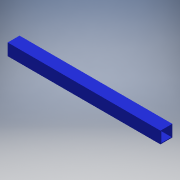
# Autodesk Inventor part: cross brace
Saved by Autodesk Inventor 2017 SP1 (Build 210196100, 196)
## iProperties
Created: 2018-01-26
Part Number: cross brace
Material: Aluminum 6061
Document SubType Name: Modeling
Designer: Ben
Density: 2.7 g/cm^3
Appearance: Blue - Wall Paint - Glossy
Author: Ben
Autodesk Inventor part; units mm, degrees
ref_plane "YZ Plane" through (0, 0, 0) normal (1, 0, 0) x (0, 1, 0)
ref_plane "XZ Plane" through (0, 0, 0) normal (0, 1, 0) x (-1, 0, 0)
ref_plane "XY Plane" through (0, 0, 0) normal (0, 0, 1) x (1, 0, 0)
sketch "Sketch1" plane through (0, 0, 0) normal (1, 0, 0) x (0, 1, 0)
  line L0 (-12.7, 12.7) -> (12.7, 12.7)
  line L1 (12.7, 12.7) -> (12.7, -12.7)
  line L2 (12.7, -12.7) -> (-12.7, -12.7)
  line L3 (-12.7, -12.7) -> (-12.7, 12.7)
  line L4 (-12.7, 12.7) -> (12.7, -12.7) construction
  line L5 (12.7, 12.7) -> (-12.7, -12.7) construction
  line L6 (-11.1125, 11.1125) -> (11.1125, 11.1125)
  line L7 (11.1125, 11.1125) -> (11.1125, -11.1125)
  line L8 (11.1125, -11.1125) -> (-11.1125, -11.1125)
  line L9 (-11.1125, -11.1125) -> (-11.1125, 11.1125)
  line L10 (-11.1125, 11.1125) -> (11.1125, -11.1125) construction
  line L11 (11.1125, 11.1125) -> (-11.1125, -11.1125) construction
  point P0 (0, 0)
  dimension "d0" = 25.4
  dimension "d1" = 1.5875
  constraints: 24 end point, 4 midpoint, 4 parallel, 3 perpendicular, 2 horizontal, 1 point on line
  measures "d0" distance of L1.end L2.end
  measures "d1" distance between parallel lines of L2 L8
extrude "Extrusion1" add sketch "Sketch1" along normal mid plane 311.15
body "Solid1"
